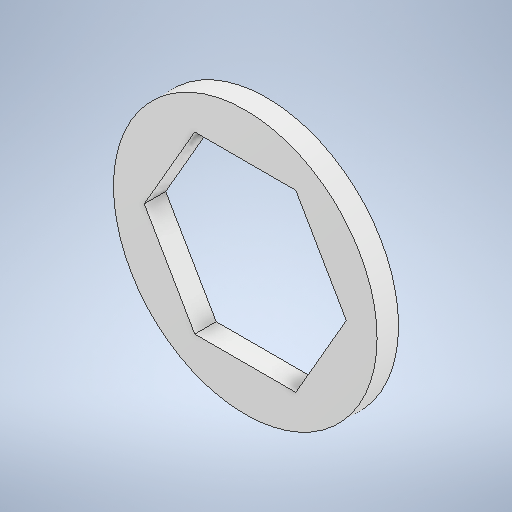
# Autodesk Inventor part: WCP-0787-01
Saved by Autodesk Inventor 2025.1 (Build 291241020, 241B)
## iProperties
Created: 2024-10-06
Part Number: WCP-0787-01
Material: PVC-Piping
Document SubType Name: Modeling
Designer: xmand
Density: 1.4 g/cm^3
Appearance: Smooth - White
Author: xmand
Autodesk Inventor part; units mm, degrees
ref_plane "YZ Plane" through (0, 0, 0) normal (1, 0, 0) x (0, 1, 0)
ref_plane "XZ Plane" through (0, 0, 0) normal (0, 1, 0) x (-1, 0, 0)
ref_plane "XY Plane" through (0, 0, 0) normal (0, 0, 1) x (1, 0, 0)
sketch "Sketch1" plane through (0, 0, 0) normal (0, 0, 1) x (1, 0, 0)
  circle A0 centre (0, 0) radius 9.7536
  line L0 (3.7395, -6.477) -> (-3.7395, -6.477)
  line L1 (-3.7395, -6.477) -> (-7.479, 0)
  line L2 (-7.479, 0) -> (-3.7395, 6.477)
  line L3 (-3.7395, 6.477) -> (3.7395, 6.477)
  line L4 (3.7395, 6.477) -> (7.479, 0)
  line L5 (7.479, 0) -> (3.7395, -6.477)
  dimension "d0" = 19.5072
  dimension "d1" = 12.954
  constraints: 12 end point, 2 coincident, 1 centre point, 1 horizontal, 13 other
  measures "d0" diameter of A0
  measures "d1" distance between parallel lines of L0 L3
extrude "Extrusion1" add sketch "Sketch1" along normal mid plane 1.5875
body "Solid1"
